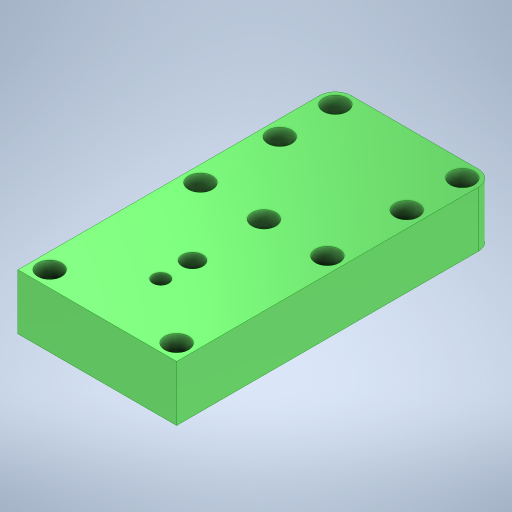
# Autodesk Inventor part: Nắp hộp piston
Saved by Autodesk Inventor 2023 (Build 270158000, 158)
## iProperties
Created: 2023-10-06
Part Number: Nắp hộp piston
Material: Iron, Gray
Document SubType Name: Modeling
Designer: huy20
Density: 7.15 g/cm^3
Appearance: Iron Gray
Author: huy20
Autodesk Inventor part; units mm, degrees
ref_plane "XZ Plane" through (0, 0, 0) normal (0, 1, 0) x (-1, 0, 0)
ref_plane "XY Plane" through (0, 0, 0) normal (0, 0, 1) x (1, 0, 0)
sketch "Sketch2" plane through (0, 0, 0) normal (0, 0, 1) x (1, 0, 0)
  line L0 (0, 0) -> (20, 0)
  line L1 (20, 0) -> (20, 7)
  line L2 (20, 7) -> (0, 7)
  line L3 (0, 7) -> (0, 0)
  dimension "d0" = 20
  dimension "d1" = 7
  constraints: 8 end point, 2 parallel, 1 horizontal, 1 perpendicular
  measures "d0" distance of L1.end L2.end
  measures "d1" distance of L0.end L1.end
extrude "Extrusion1" add sketch "Sketch2" along normal blind 40
ref_plane "Work Plane1" through (10, 0, 0) normal (1, 0, 0) x (0, 1, 0)
sketch "Sketch3" plane through (10, 0, 0) normal (1, 0, 0) x (0, 1, 0)
  line L0 (7, 40) -> (0, 40) construction
  line L1 (0, 40) -> (0, 30) construction
  line L2 (0, 0) -> (0, 40) construction
  line L3 (0, 30) -> (2, 30) construction
  line L4 (0, 30) -> (0, 23)
  line L5 (0, 23) -> (0.5, 23)
  line L6 (0, 30) -> (2, 30)
  arc A0 (0.5, 23) -> (1.333, 26.4822) centre (-72.4911, 42.3017) ccw
  line L7 (2, 30) -> (2, 26.4822)
  line L8 (2, 26.4822) -> (1.333, 26.4822)
  dimension "d4" = 10
  dimension "d5" = 2
  dimension "d6" = 7
  dimension "d9" = 0.5
  dimension "d10" = 75.5
  constraints: 14 end point, 2 perpendicular, 2 point on circle, 2 point on line, 1 centre point, 1 collinear, 1 horizontal
  measures "d4" distance of L0.end L1.end
  measures "d5" distance of L1.end L3.end
  measures "d6" distance of L1.end L4.end
  measures "d9" distance of L4.end L5.end
  measures "d10" radius of A0
revolve "Revolution1" cut sketch "Sketch3" angle 360 about axis through (10, 0, 30) along (0, 1, 0)
sketch "Sketch5" plane through (10, 2, 30) normal (0, -1, 0) x (1, 0, 0)
  circle A0 centre (0, 0) radius 3.5178 projected
  circle A1 centre (0, 2) radius 1
  circle A2 centre (0, -2) radius 1
  line L0 (1.4669, 0) -> (-1.3764, 0) construction
  point P0 (-10, -30)
  dimension "d11" = 2
  dimension "d12" = 2
  dimension "d13" = 2
  dimension "d14" = 2
  constraints: 2 centre point, 2 end point, 1 coincident, 1 horizontal
  measures "d11" diameter of A1
  measures "d12" diameter of A2
  measures "d13" distance from line of L0 A2.centre
  measures "d14" distance from line of L0 A1.centre
hole "Hole1" at (10, 2, 32) direction (0, 1, 0) diameter 2 depth 10 countersink diameter 2.5 countersink angle 60 clearance for "Flat Head Machine Screw (82)" size "#0" standard "Ansi Unified Screw Threads"
sketch "Sketch6" plane through (10, 2, 30) normal (0, -1, 0) x (1, 0, 0)
  line L0 (0, 0) -> (1.9071, 0) construction
  circle A0 centre (0, -2) radius 1
  point P0 (-10, -30)
  dimension "d22" = 2
  dimension "d23" = 2
  constraints: 2 end point, 1 centre point, 1 horizontal
  measures "d22" diameter of A0
  measures "d23" distance from line of L0 A0.centre
extrude "Extrusion2" cut sketch "Sketch6" against normal blind 40
sketch "Sketch7" plane through (10, 0, 0) normal (1, 0, 0) x (0, 1, 0)
  line L0 (2, 27) -> (2, 29) construction
  line L1 (2, 28) -> (3.2187, 28) construction
  line L2 (2.5, 26.7113) -> (2, 27)
  line L3 (2, 27) -> (2, 29) construction
  line L4 (2, 27) -> (2.7064, 27) construction
  line L5 (2, 29) -> (2.7329, 29) construction
  line L6 (2, 29) -> (7, 29) projected
  line L7 (2, 28) -> (2, 27)
  line L8 (2.5, 26.7113) -> (7.9836, 26.7113)
  line L9 (2, 28) -> (7.9836, 28)
  line L10 (8.4909, 28) -> (8.4909, 26.7113)
  line L11 (8.4909, 26.7113) -> (7.9836, 26.7113)
  line L12 (7.9836, 28) -> (8.4909, 28)
  point P0 (0, 0)
  point P1 (2.5, 28)
  dimension "d26" = 30
  constraints: 20 end point, 2 perpendicular, 2 point on line, 1 collinear, 1 horizontal, 1 midpoint
  measures "d26" angle of L2 L4
revolve "Revolution2" cut sketch "Sketch7" angle 360 about axis through (10, 2, 28) along (0, 1, 0)
fillet "Fillet1" radius 2 2 edges at (0, 3.5, 0) (20, 3.5, 0)
sketch "Sketch9" plane through (0, 7, 40) normal (0, 1, 0) x (1, 0, 0)
  circle A0 centre (2, 2) radius 0.75 projected
  circle A1 centre (2, 21) radius 0.75 projected
  circle A2 centre (2, 31) radius 0.75 projected
  circle A3 centre (2, 38) radius 0.75 projected
  circle A4 centre (18, 38) radius 0.75 projected
  circle A5 centre (18, 31) radius 0.75 projected
  circle A6 centre (18, 21) radius 0.75 projected
  circle A7 centre (10, 21) radius 0.75 projected
  point P0 (0, 40)
  point P1 (18, 2)
  constraints: 8 coincident
hole "Hole3" at (2, 7, 38) at (2, 7, 19) at (2, 7, 9) at (2, 7, 2) at (18, 7, 2) at (18, 7, 9) at (18, 7, 19) at (10, 7, 19) at (18, 7, 38) direction (0, -1, 0) diameter 2 depth 10 counterbore diameter 3 counterbore depth 2
body "Solid1"
